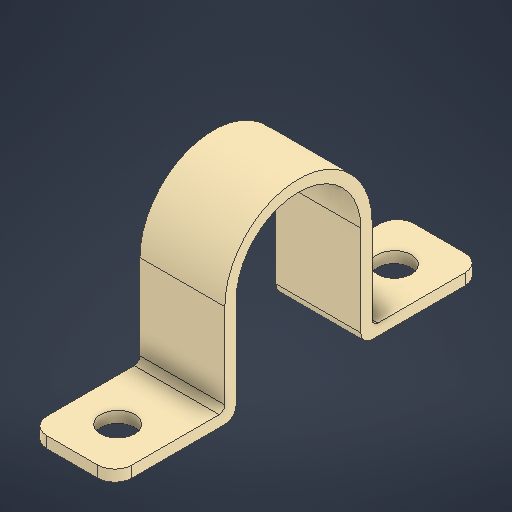
# Autodesk Inventor part: rackbracket
Saved by Autodesk Inventor 2026.2 (Build 302298010, 298A)
## iProperties
Created: 2026-07-06
Part Number: rackbracket
Material: Generic
Document SubType Name: Modeling
Designer: tasle
Density: 1 g/cm^3
Appearance: Default
Author: tasle
Autodesk Inventor part; units mm, degrees
ref_plane "YZ Plane" through (0, 0, 0) normal (1, 0, 0) x (0, 1, 0)
ref_plane "XZ Plane" through (0, 0, 0) normal (0, 1, 0) x (-1, 0, 0)
ref_plane "XY Plane" through (0, 0, 0) normal (0, 0, 1) x (1, 0, 0)
sketch "Sketch1" plane through (0, 0, 0) normal (1, 0, 0) x (0, 1, 0)
  arc A0 (0, -11) -> (0, 11) centre (0, 0) ccw
  arc A1 (0, -13) -> (0, 13) centre (0, 0) ccw
  line L0 (0, 13) -> (-16.0086, 13)
  line L1 (0, 11) -> (-18.0086, 11)
  line L2 (0, 0) -> (4.4908, 0)
  line L3 (-18.0086, 11) -> (-11, 11)
  line L4 (-16.0086, 13) -> (-16.0086, 32.4223)
  line L5 (-16.0086, 32.4223) -> (-18.0086, 32.4223)
  line L6 (-18.0086, 32.4223) -> (-18.0086, 11)
  line L7 (0, -13) -> (-16.0086, -13)
  line L8 (0, -11) -> (-18.0086, -11)
  line L9 (-18.0086, -11) -> (-11, -11)
  line L10 (-16.0086, -13) -> (-16.0086, -32.4223)
  line L11 (-16.0086, -32.4223) -> (-18.0086, -32.4223)
  line L12 (-18.0086, -32.4223) -> (-18.0086, -11)
  point P0 (-6.9282, 11)
  point P1 (-6.9282, -11)
  dimension "d0" = 22
  dimension "d1" = 2
  dimension "d2" = 22
  dimension "d12" = 18.0086
  dimension "d13" = 2
  constraints: 26 end point, 8 symmetric about line, 4 horizontal, 4 point on circle, 2 centre point, 2 parallel, 2 point on line, 1 coincident, 1 perpendicular, 1 tangent
  measures "d0" diameter of A0
  measures "d1" radial gap between concentric circles of A0 A1
  measures "d2" distance of L4.end L3.end
  measures "d12" distance from line of L12 point (0, 0)
  measures "d13" distance between parallel lines of L6 L4
extrude "Extrusion1" add sketch "Sketch1" along normal blind 15
fillet "Fillet1" radius 2 2 edges at (7.5, -18.0086, -11) (7.5, -18.0086, 11)
fillet "Fillet2" radius 1 2 edges at (7.5, -16.0086, 13) (7.5, -16.0086, -13)
fillet "Fillet3" radius 3 4 edges at (15, -17.0086, 32.4223) (0, -17.0086, 32.4223) (15, -17.0086, -32.4223) (0, -17.0086, -32.4223)
sketch "Sketch2" plane through (0, -16.0086, 14) normal (0, 1, 0) x (1, 0, 0)
  circle A0 centre (7.5, -10.4223) radius 3
  line L0 (3, -18.4223) -> (12, -18.4223) projected
  line L1 (0, 14) -> (27.6341, 14)
  circle A1 centre (7.5, 38.4223) radius 3
  dimension "d8" = 6
  dimension "d9" = 8
  constraints: 2 centre point, 2 end point, 1 horizontal, 1 symmetric about line, 1 other
  measures "d8" diameter of A0
  measures "d9" distance from line of L0 A0.centre
extrude "Extrusion2" cut sketch "Sketch2" against normal blind 15
body "Solid1"
